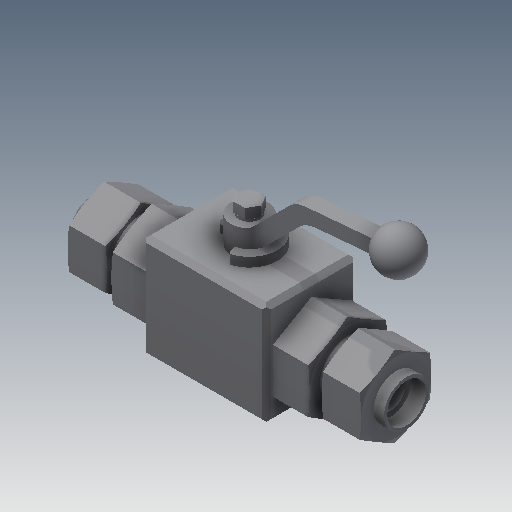
# Autodesk Inventor part: BO-KHV  15 L/NW  13 WAL602203 (offen)
Saved by Autodesk Inventor 2019.1 (Build 231200000, 200)
## iProperties
Category: PARTsolutions
Created: 2009-08-10
Part Number: BO-KHV  15 L/NW  13 WAL602203 (offen)
Catalog Web Link: www.cadenas.de
Description: BO-KHV... - Ball valve, Tube connection both ends
Document SubType Name: Modeling
Designer: PARTsolutions
Density: 1 g/cm^3
Material: Generic
Stock Number: NA
Appearance: RGB(175,175,175)
Mass: 104.117 g
Surface Area: 247.284 cm^2
Volume: 104.117 cm^3
NB: BO-KHV  15 L/NW  13 WAL602203 (offen)
NN: BO-KHV...
NT: Ball valve, Tube connection both ends
NBSYN: $TYP. $BESTNR. ($FUN.)
LINA: BO-KHV  15 L/NW  13 WAL602203 (offen)
REIHE: L
PB: 400
RO: 15
D2ZR: 11
LZR: 12.5
D1DR: 17.5
TYP: BO-KHV  15 L/NW  13
BESTNR: WAL602203
FUN: offen
B: 35
H: 40
H2: 17.5
H1: 83.0
I2: 48
I1: 84
L1: 82.0
L2: 113
L3: 121
S1: 30
S2: 27
S3: 9
R1: 107
DN: 13.000
PSTOOL: 0.010
FUNP: 1.000
BM: infotext
DOC: bo_khv.txt
KT: DUMMY
PSOL_IDENT_0: {\\partserver001.servicenet\dplatte\cadenas\23d-libs\eaton_walterscheid\boerdelrohr\05\hochdruck_kug
PSOL_IDENT_1: elhahn\bo_khv.prj},235 {VTYP=3D},{NB=BO-KHV  15 L/NW  13 WAL602203 (offen)},{LINA=BO-KHV  15 L/NW  1
PSOL_IDENT_2: 3 WAL602203 (offen)},{NN=BO-KHV...},{DATE=02.09.2008 09:49:43},{GEOMDATE=28.08.2008 12:48:00},{VERSI
PSOL_IDENT_3: ON=v040130000000},{LINEID=50},{LINESUBID=-1},{WBVAR=FUN}  {NB=BO-KHV  15 L/NW  13 WAL602203 (offen)}
PSOL_IDENT_4: ,{LINA=BO-KHV  15 L/NW  13 WAL602203 (offen)},{KT=DUMMY},{REIHE=L},{PB=400},{RO=15},{D2ZR=11},{LZR=1
PSOL_IDENT_5: 2.5},{D1DR=17.5},{TYP=BO-KHV  15 L/NW  13},{BESTNR=WAL602203},{FUN=offen},{B=35},{H=40},{H2=17.5},{H
PSOL_IDENT_6: 1=83.0},{I2=48},{I1=84},{L1=82.0},{L2=113},{L3=121},{S1=30},{S2=27},{S3=9},{R1=107},{DN=13.000},{PST
PSOL_IDENT_7: OOL=0.010},{FUNP=1},{BM=infotext},{DOC=bo_khv.txt}
Title: Purchased Part
Author: Cadenas PARTsolutions
Comments: Ball valve, Tube connection both ends
Revision Number: A
Autodesk Inventor part; units mm, degrees
ref_plane "YZ Plane" through (0, 0, 0) normal (1, 0, 0) x (0, 1, 0)
ref_plane "XZ Plane" through (0, 0, 0) normal (0, 1, 0) x (-1, 0, 0)
ref_plane "XY Plane" through (0, 0, 0) normal (0, 0, 1) x (1, 0, 0)
sketch "Skizze_1" plane through (0, 0, 0) normal (1, 0, 0) x (0, 1, 0)
  line L0 (-15.75, 17.5) -> (-17.5, 15.75)
  line L1 (-17.5, 15.75) -> (-17.5, -15.75)
  line L2 (-17.5, -15.75) -> (-15.75, -17.5)
  line L3 (-15.75, -17.5) -> (20.75, -17.5)
  line L4 (20.75, -17.5) -> (22.5, -15.75)
  line L5 (22.5, -15.75) -> (22.5, 15.75)
  line L6 (22.5, 15.75) -> (20.75, 17.5)
  line L7 (20.75, 17.5) -> (-15.75, 17.5)
  constraints: 16 end point
extrude "Extrusion1" add sketch "Skizze_1" along normal mid plane 48
sketch "Skizze_2" plane through (0, 0, 0) normal (0, 0, 1) x (1, 0, 0)
  line L0 (-48, -27.5) -> (48, -27.5)
  line L1 (48, -27.5) -> (48, 52.5)
  line L2 (48, 52.5) -> (-48, 52.5)
  line L3 (-48, 52.5) -> (-48, -27.5)
  line L4 (-24, -15.75) -> (-22.25, -17.5)
  line L5 (-22.25, -17.5) -> (22.25, -17.5)
  line L6 (22.25, -17.5) -> (24, -15.75)
  line L7 (24, -15.75) -> (24, 20.75)
  line L8 (24, 20.75) -> (22.25, 22.5)
  line L9 (22.25, 22.5) -> (-22.25, 22.5)
  line L10 (-22.25, 22.5) -> (-24, 20.75)
  line L11 (-24, 20.75) -> (-24, -15.75)
  constraints: 24 end point
extrude "Extrusion2" cut sketch "Skizze_2" along normal mid plane 35
sketch "Skizze_3" plane through (0, 0, 0) normal (0, 1, 0) x (-1, 0, 0)
  line L0 (48, -35) -> (48, 35)
  line L1 (48, 35) -> (-48, 35)
  line L2 (-48, 35) -> (-48, -35)
  line L3 (-48, -35) -> (48, -35)
  line L4 (24, -15.75) -> (24, 15.75)
  line L5 (24, 15.75) -> (22.25, 17.5)
  line L6 (22.25, 17.5) -> (-22.25, 17.5)
  line L7 (-22.25, 17.5) -> (-24, 15.75)
  line L8 (-24, 15.75) -> (-24, -15.75)
  line L9 (-24, -15.75) -> (-22.25, -17.5)
  line L10 (-22.25, -17.5) -> (22.25, -17.5)
  line L11 (22.25, -17.5) -> (24, -15.75)
  constraints: 24 end point
extrude "Extrusion3" cut sketch "Skizze_3" along normal mid plane 80
sketch "Skizze_4" plane through (0, 0, 0) normal (0, 0, 1) x (1, 0, 0)
  line L0 (38.1818, 0) -> (24, 0)
  line L1 (24, 0) -> (24, 7.5)
  line L2 (24, 7.5) -> (24.02, 7.5)
  line L3 (24.02, 7.5) -> (24.02, 18)
  line L4 (24.02, 18) -> (37.378, 18)
  line L5 (37.378, 18) -> (38.1818, 15)
  line L6 (38.1818, 15) -> (38.1818, 0)
  line L7 (38.1818, 0) -> (24, 0)
  constraints: 16 end point
sketch "Skizze_6" plane through (0, 0, 0) normal (0, 0, 1) x (1, 0, 0)
  line L0 (-24, 0) -> (-38.1818, 0)
  line L1 (-38.1818, 0) -> (-38.1818, 15)
  line L2 (-38.1818, 15) -> (-37.378, 18)
  line L3 (-37.378, 18) -> (-24.02, 18)
  line L4 (-24.02, 18) -> (-24.02, 7.5)
  line L5 (-24.02, 7.5) -> (-24, 7.5)
  line L6 (-24, 7.5) -> (-24, 0)
  line L7 (-24, 0) -> (-38.1818, 0)
  constraints: 16 end point
revolve "Revolution1" add sketch "Skizze_6" angle 360 about axis through (-24, 0, 0) along (1, 0, 0)
sketch "Skizze_8" plane through (0, 0, 0) normal (0, 0, 1) x (1, 0, 0)
  line L0 (60.5, 0) -> (-60.5, 0)
  line L1 (-60.5, 0) -> (-60.5, 7.5)
  line L2 (-60.5, 7.5) -> (-54.5, 7.5)
  line L3 (-54.5, 7.5) -> (-54.5, 5.5)
  line L4 (-54.5, 5.5) -> (-42, 5.5)
  line L5 (-42, 5.5) -> (-42, 6.25)
  line L6 (-42, 6.25) -> (42, 6.25)
  line L7 (42, 6.25) -> (42, 5.5)
  line L8 (42, 5.5) -> (54.5, 5.5)
  line L9 (54.5, 5.5) -> (54.5, 7.5)
  line L10 (54.5, 7.5) -> (60.5, 7.5)
  line L11 (60.5, 7.5) -> (60.5, 0)
  line L12 (60.5, 0) -> (-60.5, 0)
  constraints: 26 end point
sketch "Skizze_5" plane through (38.1818, 0, 0) normal (1, 0, 0) x (0, 0, -1)
  line L0 (-45, 25.9808) -> (-45, -25.9808)
  line L1 (-45, -25.9808) -> (0, -51.9615)
  line L2 (0, -51.9615) -> (45, -25.9808)
  line L3 (45, -25.9808) -> (45, 25.9808)
  line L4 (45, 25.9808) -> (0, 51.9615)
  line L5 (0, 51.9615) -> (-45, 25.9808)
  line L6 (-15, 8.6603) -> (-15, -8.6603)
  line L7 (-15, -8.6603) -> (0, -17.3205)
  line L8 (0, -17.3205) -> (15, -8.6603)
  line L9 (15, -8.6603) -> (15, 8.6603)
  line L10 (15, 8.6603) -> (0, 17.3205)
  line L11 (0, 17.3205) -> (-15, 8.6603)
  constraints: 24 end point
sketch "Skizze_7" plane through (-38.1818, 0, 0) normal (1, 0, 0) x (0, 0, -1)
  line L0 (-45, 25.9808) -> (-45, -25.9808)
  line L1 (-45, -25.9808) -> (0, -51.9615)
  line L2 (0, -51.9615) -> (45, -25.9808)
  line L3 (45, -25.9808) -> (45, 25.9808)
  line L4 (45, 25.9808) -> (0, 51.9615)
  line L5 (0, 51.9615) -> (-45, 25.9808)
  line L6 (-15, 8.6603) -> (-15, -8.6603)
  line L7 (-15, -8.6603) -> (0, -17.3205)
  line L8 (0, -17.3205) -> (15, -8.6603)
  line L9 (15, -8.6603) -> (15, 8.6603)
  line L10 (15, 8.6603) -> (0, 17.3205)
  line L11 (0, 17.3205) -> (-15, 8.6603)
  constraints: 24 end point
extrude "Extrusion4" cut sketch "Skizze_7" along normal blind 14.1718
sketch "Skizze_10" plane through (0, 0, 0) normal (0, 0, 1) x (1, 0, 0)
  line L0 (-9, 26.1) -> (-9, 22.5)
  line L1 (-9, 22.5) -> (-10.8, 22.5)
  line L2 (-10.8, 22.5) -> (-10.8, 25.6)
  line L3 (-10.8, 25.6) -> (-10.3, 26.1)
  line L4 (-10.3, 26.1) -> (-9, 26.1)
  line L5 (-9, 26.1) -> (-9, 22.5)
  constraints: 12 end point
revolve "Revolution2" add sketch "Skizze_10" angle 360 about axis through (-9, 26.1, 0) along (0, 1, 0)
sketch "Skizze_12" plane through (0, 22.5, 0) normal (0, 1, 0) x (1, 0, 0)
  arc A0 (-10.2504, 3.4013) -> (-9.5178, 2.11) centre (-9.3013, 3.0863) ccw
  line L0 (-9.5178, 2.11) -> (-7.7491, 1.7179)
  arc A1 (-6.9699, 0.6489) -> (-7.7491, 1.7179) centre (-7.9655, 0.7416) ccw
  arc A2 (-6.9699, 0.6489) -> (0.6489, -6.9699) centre (0, 0) ccw
  arc A3 (1.7179, -7.7491) -> (0.6489, -6.9699) centre (0.7416, -7.9655) ccw
  line L1 (1.7179, -7.7491) -> (2.11, -9.5178)
  arc A4 (2.11, -9.5178) -> (3.4013, -10.2504) centre (3.0863, -9.3013) ccw
  arc A5 (3.4013, -10.2504) -> (-10.2504, 3.4013) centre (0, 0) ccw
  constraints: 12 point on circle, 6 centre point, 4 end point
extrude "Extrusion5" add sketch "Skizze_12" along normal mid plane 7.2
sketch "Skizze_14" plane through (0, 0, 0) normal (0, 0, 1) x (1, 0, 0)
  line L0 (-7.22, 26.1) -> (5.1089, 26.1)
  arc A0 (5.1089, 26.1) -> (8.6445, 27.5645) centre (5.1089, 31.1) ccw
  line L1 (8.6445, 27.5645) -> (22.0454, 40.9654)
  arc A1 (28.2449, 43.8563) -> (22.0454, 40.9654) centre (29.1165, 33.8943) ccw
  line L2 (28.2449, 43.8563) -> (57.2953, 46.3979)
  line L3 (57.2953, 46.3979) -> (57.2953, 51.8328)
  line L4 (57.2953, 51.8328) -> (24.4223, 48.9568)
  arc A2 (24.4223, 48.9568) -> (18.2228, 46.0659) centre (25.2939, 38.9948) ccw
  line L5 (18.2228, 46.0659) -> (5.7658, 33.6089)
  arc A3 (4.3516, 33.0231) -> (5.7658, 33.6089) centre (4.3516, 35.0231) ccw
  line L6 (4.3516, 33.0231) -> (-7.22, 33.0231)
  line L7 (-7.22, 33.0231) -> (-7.22, 26.1)
  constraints: 16 end point, 8 point on circle, 4 centre point
sketch "Skizze_15" plane through (0, 26.09, 0) normal (0, 1, 0) x (1, 0, 0)
  line L0 (-35.6667, 18) -> (-35.6667, -18)
  line L1 (-35.6667, -18) -> (124.8333, -18)
  line L2 (124.8333, -18) -> (124.8333, -3)
  line L3 (124.8333, -3) -> (8.743, -3)
  arc A0 (8.743, -3) -> (5.6205, -4.5) centre (8.743, -7) ccw
  arc A1 (5.6205, 4.5) -> (5.6205, -4.5) centre (0, 0) ccw
  arc A2 (5.6205, 4.5) -> (8.743, 3) centre (8.743, 7) ccw
  line L4 (8.743, 3) -> (124.8333, 3)
  line L5 (124.8333, 3) -> (124.8333, 18)
  line L6 (124.8333, 18) -> (-35.6667, 18)
  constraints: 14 end point, 6 point on circle, 3 centre point
sketch "Skizze_16" plane through (0, 0, 0) normal (0, 0, 1) x (1, 0, 0)
  line L0 (57.374, 57.5268) -> (57.374, 41.222)
  arc A0 (57.374, 57.5268) -> (57.374, 41.222) centre (57.374, 49.3744) ccw
  line L1 (57.374, 57.5268) -> (57.374, 41.222)
  constraints: 4 end point, 2 point on circle, 1 centre point
sketch "Skizze_20" plane through (0, 0, 0) normal (0, 0, 1) x (1, 0, 0)
  line L0 (0, 33.0231) -> (0, 33.9231)
  line L1 (0, 33.9231) -> (4.0909, 33.9231)
  line L2 (4.0909, 33.9231) -> (4.0909, 33.0231)
  line L3 (4.0909, 33.0231) -> (0, 33.0231)
  line L4 (0, 33.0231) -> (0, 33.9231)
  constraints: 10 end point
sketch "Skizze_21" plane through (0, 0, 0) normal (0, 0, 1) x (1, 0, 0)
  line L0 (0, 33.9231) -> (0, 37.9231)
  line L1 (0, 37.9231) -> (4, 37.9231)
  line L2 (4, 37.9231) -> (4.8, 37.7087)
  line L3 (4.8, 37.7087) -> (4.8, 34.1374)
  line L4 (4.8, 34.1374) -> (4, 33.9231)
  line L5 (4, 33.9231) -> (0, 33.9231)
  line L6 (0, 33.9231) -> (0, 37.9231)
  constraints: 14 end point
revolve "Revolution3" add sketch "Skizze_4" angle 360 about axis through (38.1818, 0, 0) along (1, 0, 0)
extrude "Extrusion6" cut sketch "Skizze_5" against normal blind 14.1718
sketch "Skizze_22" plane through (0, 0, 0) normal (0, 0, 1) x (1, 0, 0)
  line L0 (60.5, 0) -> (0, 0)
  line L1 (-60.5, 0) -> (-60.5, 8.75)
  line L2 (-60.5, 8.75) -> (-56.5, 8.75)
  line L3 (-56.5, 8.75) -> (-56.5, 13.5)
  line L4 (-56.5, 13.5) -> (-55.7765, 16.2)
  line L5 (-55.7765, 16.2) -> (-42, 16.2)
  line L6 (-42, 16.2) -> (-41.2765, 13.5)
  line L7 (-41.2765, 13.5) -> (-41.2765, 12.2727)
  line L8 (-41.2765, 12.2727) -> (-40, 12.2727)
  line L9 (-40, 12.2727) -> (-39.2061, 11.4788)
  arc A0 (-39.2061, 11.4788) -> (-38.1818, 11.9031) centre (-38.7818, 11.9031) ccw
  line L10 (-38.1818, 11.9031) -> (-38.1818, 14.2857)
  line L11 (-38.1818, 14.2857) -> (38.1818, 14.2857)
  line L12 (38.1818, 14.2857) -> (38.1818, 11.9031)
  arc A1 (38.1818, 11.9031) -> (39.2061, 11.4788) centre (38.7818, 11.9031) ccw
  line L13 (39.2061, 11.4788) -> (40, 12.2727)
  line L14 (40, 12.2727) -> (41.2765, 12.2727)
  line L15 (41.2765, 12.2727) -> (41.2765, 13.5)
  line L16 (41.2765, 13.5) -> (42, 16.2)
  line L17 (42, 16.2) -> (55.7765, 16.2)
  line L18 (55.7765, 16.2) -> (56.5, 13.5)
  line L19 (56.5, 13.5) -> (56.5, 8.75)
  line L20 (56.5, 8.75) -> (60.5, 8.75)
  line L21 (60.5, 8.75) -> (60.5, 0)
  line L22 (60.5, 0) -> (-60.5, 0)
  constraints: 46 end point, 4 point on circle, 2 centre point
revolve "Revolution4" add sketch "Skizze_22" angle 360 about axis through (60.5, 0, 0) along (1, 0, 0)
sketch "Skizze_26" plane through (-56.5, 0, 0) normal (1, 0, 0) x (0, 0, -1)
  line L0 (-27, 15.5885) -> (-27, -15.5885)
  line L1 (-27, -15.5885) -> (0, -31.1769)
  line L2 (0, -31.1769) -> (27, -15.5885)
  line L3 (27, -15.5885) -> (27, 15.5885)
  line L4 (27, 15.5885) -> (0, 31.1769)
  line L5 (0, 31.1769) -> (-27, 15.5885)
  line L6 (-13.5, 7.7942) -> (-13.5, -7.7942)
  line L7 (-13.5, -7.7942) -> (0, -15.5885)
  line L8 (0, -15.5885) -> (13.5, -7.7942)
  line L9 (13.5, -7.7942) -> (13.5, 7.7942)
  line L10 (13.5, 7.7942) -> (0, 15.5885)
  line L11 (0, 15.5885) -> (-13.5, 7.7942)
  constraints: 24 end point
extrude "Extrusion7" cut sketch "Skizze_26" along normal mid plane 36.6164
sketch "Skizze_27" plane through (56.5, 0, 0) normal (1, 0, 0) x (0, 0, -1)
  line L0 (-27, 15.5885) -> (-27, -15.5885)
  line L1 (-27, -15.5885) -> (0, -31.1769)
  line L2 (0, -31.1769) -> (27, -15.5885)
  line L3 (27, -15.5885) -> (27, 15.5885)
  line L4 (27, 15.5885) -> (0, 31.1769)
  line L5 (0, 31.1769) -> (-27, 15.5885)
  line L6 (-13.5, 7.7942) -> (-13.5, -7.7942)
  line L7 (-13.5, -7.7942) -> (0, -15.5885)
  line L8 (0, -15.5885) -> (13.5, -7.7942)
  line L9 (13.5, -7.7942) -> (13.5, 7.7942)
  line L10 (13.5, 7.7942) -> (0, 15.5885)
  line L11 (0, 15.5885) -> (-13.5, 7.7942)
  constraints: 24 end point
extrude "Extrusion8" cut sketch "Skizze_27" along normal mid plane 36.6164
revolve "Revolution5" cut sketch "Skizze_8" angle 360 about axis through (60.5, 0, 0) along (1, 0, 0)
extrude "Extrusion9" add sketch "Skizze_14" along normal mid plane 14.4
extrude "Extrusion10" cut sketch "Skizze_15" along normal blind 83
revolve "Revolution6" add sketch "Skizze_20" angle 360 about axis through (0, 33.0231, 0) along (0, -1, 0)
revolve "Revolution7" add sketch "Skizze_21" angle 360 about axis through (0, 33.9231, 0) along (0, -1, 0)
sketch "Skizze_9" plane through (0, 37.9231, 0) normal (0, 1, 0) x (1, 0, 0)
  line L0 (-5.7735, 0) -> (-2.8868, -5)
  line L1 (-2.8868, -5) -> (2.8868, -5)
  line L2 (2.8868, -5) -> (5.7735, 0)
  line L3 (5.7735, 0) -> (2.8868, 5)
  line L4 (2.8868, 5) -> (-2.8868, 5)
  line L5 (-2.8868, 5) -> (-5.7735, 0)
  line L6 (-4.6188, 0) -> (-2.3094, -4)
  line L7 (-2.3094, -4) -> (2.3094, -4)
  line L8 (2.3094, -4) -> (4.6188, 0)
  line L9 (4.6188, 0) -> (2.3094, 4)
  line L10 (2.3094, 4) -> (-2.3094, 4)
  line L11 (-2.3094, 4) -> (-4.6188, 0)
  constraints: 24 end point
extrude "Extrusion11" cut sketch "Skizze_9" against normal blind 4
revolve "Revolution8" add sketch "Skizze_16" angle 360 about axis through (57.374, 57.5268, 0) along (0, 1, 0)
body "Solid1"
